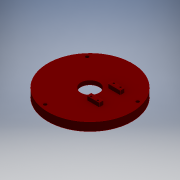
# Autodesk Inventor part: rotate_plate_3
Saved by Autodesk Inventor 2018 (Build 220112000, 112)
## iProperties
Created: 2019-01-16
Part Number: rotate_plate_3
Material: 一般
Document SubType Name: Modeling
Designer: lowyu
Density: 1 g/cm^3
Appearance: 既定
Author: lowyu
## iProperties of the stored document fix_plate_3_3D プリント.ipt
Created: 2019-01-16
Part Number: fix_plate_3_3D プリント
Material: 一般
Document SubType Name: Modeling
Designer: lowyu
Density: 1 g/cm^3
Appearance: 既定
Author: lowyu
Autodesk Inventor part; units mm, degrees
note: some values were not read from the file. Chosen so that the rebuilt part matches the saved one: second side of "押し出し3".
ref_plane "YZ Plane" through (0, 0, 0) normal (1, 0, 0) x (0, 1, 0)
ref_plane "XZ Plane" through (0, 0, 0) normal (0, 1, 0) x (-1, 0, 0)
ref_plane "XY Plane" through (0, 0, 0) normal (0, 0, 1) x (1, 0, 0)
sketch "スケッチ1" plane through (0, 0, 0) normal (0, 0, 1) x (1, 0, 0)
  circle A0 centre (0, 0) radius 50
  circle A1 centre (0, 0) radius 40
  circle A2 centre (-33.4581, 30.0925) radius 2.05
  circle A3 centre (-9.3318, -44.0218) radius 2.05
  circle A4 centre (42.7899, 13.9293) radius 2.05
  dimension "d0" = 100
  dimension "d1" = 80
  dimension "d2" = 4.1
  dimension "d4" = 45
  dimension "d7" = 360
  constraints: 5 centre point, 2 coincident, 7 other
  measures "d0" diameter of A0
  measures "d1" diameter of A1
  measures "d2" diameter of A2
  measures "d4" distance of A2.centre A1.centre
extrude "押し出し1" add sketch "スケッチ1" along normal blind 10 contours A0 | A1
sketch "スケッチ2" plane through (0, 0, 0) normal (0, 0, -1) x (-1, 0, 0)
  circle A0 centre (0, 0) radius 50
  circle A1 centre (0, 0) radius 40
  circle A2 centre (-33.4581, 30.0925) radius 2.05
  circle A3 centre (-9.3318, -44.0218) radius 2.05
  circle A4 centre (42.7899, 13.9293) radius 2.05
  dimension "d13" = 100
  dimension "d14" = 80
  dimension "d17" = 360
  constraints: 5 centre point, 2 coincident, 7 other
  measures "d13" diameter of A0
  measures "d14" diameter of A1
extrude "押し出し2" cut sketch "スケッチ2" against normal blind 5 contours A1
sketch "スケッチ3" plane through (0, 0, 5) normal (0, 0, -1) x (-1, 0, 0)
  circle A0 centre (0, 0) radius 41
  circle A1 centre (0, 0) radius 40
  dimension "d21" = 80
  dimension "d22" = 82
  constraints: 3 coincident, 2 centre point
  measures "d21" diameter of A1
  measures "d22" diameter of A0
extrude "押し出し3" cut sketch "スケッチ3" along normal blind 2
sketch "スケッチ4" plane through (0, 0, 5) normal (0, 0, -1) x (-1, 0, 0)
  circle A0 centre (0, 0) radius 35
  circle A1 centre (0, 0) radius 16
  dimension "d27" = 70
  dimension "d28" = 32
  constraints: 2 centre point, 2 coincident
  measures "d27" diameter of A0
  measures "d28" diameter of A1
extrude "押し出し4" cut sketch "スケッチ4" against normal blind 1.5
sketch "スケッチ5" plane through (0, 0, 5) normal (0, 0, -1) x (-1, 0, 0)
  circle A0 centre (0, 0) radius 11
  dimension "d31" = 22
  constraints: 1 centre point, 1 coincident
  measures "d31" diameter of A0
extrude "押し出し5" cut sketch "スケッチ5" against normal blind 5
sketch "スケッチ8" plane through (0, 0, 10) normal (0, 0, 1) x (1, 0, 0)
  circle A0 centre (0, 0) radius 11
  line L0 (0, 0) -> (3.5, 0)
  line L1 (11.5, 10) -> (11.5, 15)
  line L2 (11.5, 15) -> (26, 15)
  line L3 (11.5, 10) -> (26, 10)
  line L4 (26, 10) -> (26, 15)
  circle A1 centre (14.75, 13.5) radius 1.25
  circle A2 centre (22.75, 13.5) radius 1.25
  line L5 (-70, 0) -> (70, 0)
  line L6 (11.5, -10) -> (11.5, -15)
  line L7 (11.5, -15) -> (26, -15)
  line L8 (11.5, -10) -> (26, -10)
  line L9 (26, -10) -> (26, -15)
  circle A3 centre (14.75, -13.5) radius 1.25
  circle A4 centre (22.75, -13.5) radius 1.25
  line L10 (0, -70) -> (0, 70) projected
  line L11 (-98, 0) -> (98, 0) projected
  dimension "d54" = 5
  dimension "d55" = 14.5
  dimension "d56" = 2.5
  dimension "d57" = 3.25
  dimension "d58" = 1.5
  dimension "d59" = 2.5
  dimension "d60" = 3.25
  dimension "d64" = 27
  dimension "d65" = 11.5
  constraints: 22 end point, 6 symmetric about line, 5 centre point, 3 horizontal, 2 vertical, 1 collinear, 1 horizontal alignment, 2 other
  measures "d54" distance of L1.start L1.end
  measures "d55" distance of L1.end L2.end
  measures "d56" diameter of A1
  measures "d57" distance from line of A1.centre L1
  measures "d58" distance from line of L2 A1.centre
  measures "d59" diameter of A2
  measures "d60" distance from line of L4 A2.centre
  measures "d64" distance of A1.centre A3.centre
  measures "d65" distance between parallel lines of L1 L10
extrude "押し出し7" add sketch "スケッチ8" along normal blind 5 contours L1 L2 L4 L3 | L8 L9 L7 L6
